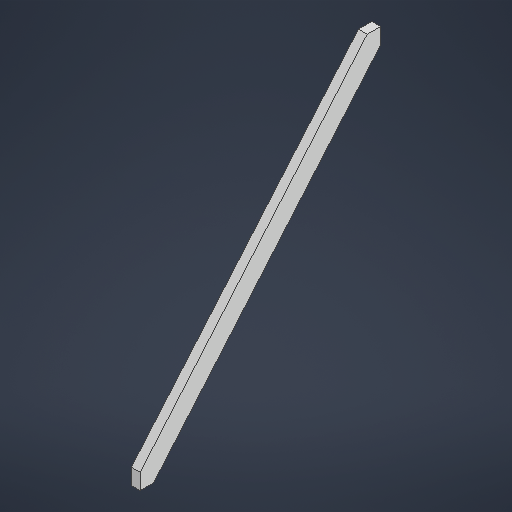
# Autodesk Inventor part: S_2x4x63.13
Saved by Autodesk Inventor 2027.1 (Build 311270010, 270A)
## iProperties
Created: 2026-08-30
Part Number: S_2x4x63.13
Material: Generic
Document SubType Name: Modeling
Designer: jorda
Density: 1 g/cm^3
Appearance: Default
Author: jorda
Autodesk Inventor part; units mm, degrees
ref_plane "YZ Plane" through (0, 0, 0) normal (1, 0, 0) x (0, 1, 0)
ref_plane "XZ Plane" through (0, 0, 0) normal (0, 1, 0) x (-1, 0, 0)
ref_plane "XY Plane" through (0, 0, 0) normal (0, 0, 1) x (1, 0, 0)
sketch "Sketch1" plane through (0, 0, 0) normal (1, 0, 0) x (0, 1, 0)
  line L0 (0, 0) -> (68.4388, 0)
  line L1 (1219.2, -1041.4) -> (1150.7612, -1041.4)
  line L2 (1150.7612, -1041.4) -> (0, -58.4581)
  line L3 (1219.2, -982.9419) -> (1219.2, -1041.4)
  line L4 (68.4388, 0) -> (1219.2, -982.9419)
  line L5 (0, -58.4581) -> (0, 0)
  constraints: 12 end point, 2 parallel, 1 horizontal, 1 perpendicular
extrude "Extrusion1" add sketch "Sketch1" along normal blind 38.1
body "Solid1"
